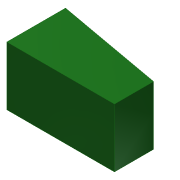
# Autodesk Inventor part: Slope 3
Saved by Autodesk Inventor 2015 SP1 (Build 190203100, 203)
## iProperties
Created: 2015-08-24
Part Number: Slope 3
Material: 一般
Document SubType Name: Modeling
Designer: nobuhiro
Density: 1 g/cm^3
Appearance: 滑らか - 濃い深緑
Author: nobuhiro
Autodesk Inventor part; units mm, degrees
ref_plane "YZ Plane" through (0, 0, 0) normal (1, 0, 0) x (0, 1, 0)
ref_plane "XZ Plane" through (0, 0, 0) normal (0, 1, 0) x (-1, 0, 0)
ref_plane "XY Plane" through (0, 0, 0) normal (0, 0, 1) x (1, 0, 0)
sketch "スケッチ1" plane through (0, 0, 0) normal (0, 0, 1) x (1, 0, 0)
  line L0 (0, 0) -> (1100, 0)
  line L1 (1100, 0) -> (1100, 400)
  line L2 (1100, 400) -> (0, 600)
  line L3 (0, 600) -> (0, 0)
  dimension "d0" = 600
  dimension "d1" = 1100
  dimension "d2" = 400
  constraints: 8 end point, 1 horizontal, 1 parallel, 1 perpendicular
  measures "d0" distance of L2.end L0.start
  measures "d1" distance of L0.start L0.end
  measures "d2" distance of L0.end L1.end
extrude "押し出し1" add sketch "スケッチ1" along normal mid plane 600
sketch "スケッチ2" plane through (0, 0, 0) normal (0, 0, 1) x (1, 0, 0)
  line L0 (1100, 400) -> (0, 600) projected
  line L1 (0, 600) -> (0, 600.1016)
  line L2 (0, 600.1016) -> (1100.0179, 400.0984)
  line L3 (1100.0179, 400.0984) -> (1100, 400)
  point P0 (0, 0)
  dimension "d5" = 0.1
  constraints: 6 end point, 1 parallel, 1 perpendicular, 1 vertical
  measures "d5" distance between parallel lines of L2 L0
extrude "押し出し2" add sketch "スケッチ2" along normal mid plane 30
